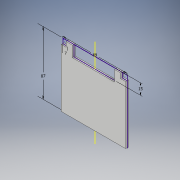
# Autodesk Inventor part: plate
Saved by Autodesk Inventor 2019.3 (Build 233278000, 278)
## iProperties
Created: 2019-06-11
Part Number: plate
Material: Generic
Document SubType Name: Modeling
Designer: Frienddo
Density: 1 g/cm^3
Appearance: Default
Author: Frienddo
Autodesk Inventor part; units mm, degrees
ref_plane "YZ Plane" through (0, 0, 0) normal (1, 0, 0) x (0, 1, 0)
ref_plane "XZ Plane" through (0, 0, 0) normal (0, 1, 0) x (-1, 0, 0)
ref_plane "XY Plane" through (0, 0, 0) normal (0, 0, 1) x (1, 0, 0)
sketch "Sketch1" plane through (0, 0, 0) normal (0, 0, 1) x (1, 0, 0)
  line L0 (44.5, -43.5) -> (-44.5, -43.5)
  line L1 (-44.5, -43.5) -> (-44.5, 43.5)
  line L2 (-44.5, 43.5) -> (44.5, 43.5)
  line L3 (44.5, 43.5) -> (44.5, -43.5)
  line L4 (44.5, -43.5) -> (-44.5, 43.5) construction
  line L5 (-44.5, -43.5) -> (44.5, 43.5) construction
  line L6 (-29.1552, 43.5) -> (29.1552, 43.5)
  line L7 (29.1552, 43.5) -> (29.1552, 28.5)
  line L8 (29.1552, 28.5) -> (-29.1552, 28.5)
  line L9 (-29.1552, 28.5) -> (-29.1552, 43.5)
  line L10 (-34.5, -43.5) -> (35.5, -43.5)
  line L11 (0, 60.9) -> (0, -60.9) projected
  line L12 (-44.5, 43.5) -> (-37.5, 43.5)
  line L13 (-37.5, 43.5) -> (-37.5, 36.6573)
  line L14 (-37.5, 36.6573) -> (-44.5, 36.6573)
  line L15 (-44.5, 36.6573) -> (-44.5, 43.5)
  line L16 (44.5, 43.5) -> (37.5, 43.5)
  line L17 (37.5, 43.5) -> (37.5, 36.6573)
  line L18 (37.5, 36.6573) -> (44.5, 36.6573)
  line L19 (44.5, 36.6573) -> (44.5, 43.5)
  point P0 (0, 0)
  dimension "d0" = 89
  dimension "d1" = 87
  dimension "d2" = 15
  dimension "d6" = 7
  constraints: 38 end point, 8 parallel, 7 point on line, 5 horizontal, 4 perpendicular, 2 midpoint
  measures "d0" distance of L1.end L2.end
  measures "d1" distance of L0.end L1.end
  measures "d2" distance of L6.end L7.end
  measures "d6" distance of L13.end L14.end
extrude "Extrusion1" add sketch "Sketch1" along normal mid plane 4 contours L0 L11 L8 L7 L2 L17 L18 L3 | L18 L17 L2 L3 | L0 L1 L14 L13 L2 L9 L8 L11 | L1 L2 L13 L14
extrude "Extrusion2" cut sketch "Sketch1" along normal mid plane 4 contours L18 L17 L2 L3 | L1 L2 L13 L14
body "Solid1"
